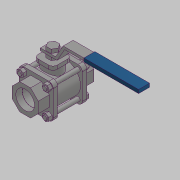
# Autodesk Inventor part: MANUAL THREADED BALL VALVE DN32 S235
Saved by Autodesk Inventor 2017 (Build 210142000, 142)
## iProperties
Created: 2017-11-25
Part Number: MANUAL THREADED BALL VALVE DN32 S235
Material: S235
Document SubType Name: Modeling
Designer: Demarec
Density: 7.85 g/cm^3
Appearance: Plate(1)
Description: BELVEN BV3
Author: Demarec
Autodesk Inventor part; units mm, degrees
ref_plane "YZ Plane" through (0, 0, 0) normal (1, 0, 0) x (0, 1, 0)
ref_plane "XZ Plane" through (0, 0, 0) normal (0, 1, 0) x (-1, 0, 0)
sketch "Sketch3" plane through (0, 0, 0) normal (0, 1, 0) x (-1, 0, 0)
  line L0 (-10.3553, 25) -> (10.3553, 25)
  line L1 (10.3553, 25) -> (25, 10.3553)
  line L2 (25, 10.3553) -> (25, -10.3553)
  line L3 (25, -10.3553) -> (10.3553, -25)
  line L4 (10.3553, -25) -> (-10.3553, -25)
  line L5 (-10.3553, -25) -> (-25, -10.3553)
  line L6 (-25, -10.3553) -> (-25, 10.3553)
  line L7 (-25, 10.3553) -> (-10.3553, 25)
  circle A0 centre (0, 0) radius 27.0598
  line L8 (24.375, -32.5) -> (-24.375, -32.5)
  line L9 (-32.5, -24.375) -> (-32.5, 24.375)
  line L10 (-24.375, 32.5) -> (24.375, 32.5)
  line L11 (32.5, 24.375) -> (32.5, -24.375)
  line L12 (32.5, -32.5) -> (-32.5, 32.5) construction
  line L13 (-32.5, -32.5) -> (32.5, 32.5) construction
  circle A1 centre (0, 0) radius 25
  arc A2 (32.5, 24.375) -> (24.375, 32.5) centre (24.375, 24.375) ccw
  arc A3 (-24.375, 32.5) -> (-32.5, 24.375) centre (-24.375, 24.375) ccw
  arc A4 (-32.5, -24.375) -> (-24.375, -32.5) centre (-24.375, -24.375) ccw
  arc A5 (24.375, -32.5) -> (32.5, -24.375) centre (24.375, -24.375) ccw
  circle A6 centre (0, 0) radius 17.5
  circle A7 centre (24.375, 24.375) radius 4
  circle A8 centre (0, 0) radius 29.0598
  dimension "oSW" = 50
  dimension "oFlangeW" = 65
  dimension "d2" = 8.125
  dimension "oIntDia" = 35
  dimension "oMbolt" = 8
  dimension "d16" = 2
  constraints: 28 end point, 9 tangent, 8 centre point, 8 point on circle, 8 point on line, 5 coincident, 3 equal radius, 2 horizontal, 2 midpoint, 2 parallel, 2 perpendicular, 20 other
  measures "oSW" distance between parallel lines of L6 L2
  measures "oFlangeW" distance of L12.start L13.start
  measures "d2" radius of A2
  measures "oIntDia" diameter of A6
  measures "oMbolt" diameter of A7
extrude "Extrusion1" add sketch "Sketch3" along normal mid plane 106 contours L0 A1 L7 | L0 L1 A1 | A1 | A1 L6 L7 | L1 L2 A1 | A1 L5 L6 | L2 L3 A1 | A1 L4 L5 | L3 L4 A1
extrude "Extrusion2" add sketch "Sketch3" along normal mid plane 64 contours A0 L0 | L7 A0 | A0 L1 | L6 A0 | A0 L2 | L5 A0 | L4 A0 | A0 L3 | L8 A4 L9 A3 L10 A2 L11 A5 | A7 | A8
extrude "Extrusion3" cut sketch "Sketch3" along normal mid plane 47 contours L8 A4 L9 A3 L10 A2 L11 A5 | A7
extrude "Extrusion4" add sketch "Sketch3" along normal mid plane 80 contours A7
sketch "Sketch4" plane through (0, -32, 0) normal (0, -1, 0) x (1, 0, 0)
  circle A0 centre (-24.375, 24.375) radius 4 projected
  line L0 (-20.9109, 18.375) -> (-27.8391, 18.375)
  line L1 (-27.8391, 18.375) -> (-31.3032, 24.375)
  line L2 (-31.3032, 24.375) -> (-27.8391, 30.375)
  line L3 (-27.8391, 30.375) -> (-20.9109, 30.375)
  line L4 (-20.9109, 30.375) -> (-17.4468, 24.375)
  line L5 (-17.4468, 24.375) -> (-20.9109, 18.375)
  point P0 (0, 0)
  dimension "d13" = 12
  constraints: 12 end point, 1 coincident, 1 horizontal, 13 other
  measures "d13" distance between parallel lines of L0 L3
extrude "Extrusion5" add sketch "Sketch4" along normal blind 6.4
sketch "Sketch10" plane through (0, 53, 0) normal (0, 1, 0) x (1, 0, 0)
  circle A0 centre (0, 0) radius 17.5 projected
  circle A1 centre (0, 0) radius 17.75
  dimension "d44" = 0.25
  constraints: 1 centre point
  measures "d44" radial gap between concentric circles of A0 A1
extrude "Extrusion11" cut sketch "Sketch10" against normal blind 12
mirror "Mirror1" about plane through (0, 0, 0) normal (0, 1, 0) of "Extrusion5", "Extrusion11"
pattern_circular "Circular Pattern1" count 4 over 360 about axis through (0, 0, 0) along (0, 1, 0) of "Extrusion5", "Extrusion4", "Mirror1"
ref_plane "Work Plane1" through (0, 0, 45) normal (0, 0, 1) x (1, 0, 0)
sketch "Sketch5" plane through (0, 0, 45) normal (0, 0, 1) x (1, 0, 0)
  line L0 (-9.875, -18) -> (9.875, -18)
  line L1 (18, -9.875) -> (18, 9.875)
  line L2 (9.875, 18) -> (-9.875, 18)
  line L3 (-18, 9.875) -> (-18, -9.875)
  line L4 (-18, -18) -> (18, 18) construction
  line L5 (18, -18) -> (-18, 18) construction
  arc A0 (-18, -9.875) -> (-9.875, -18) centre (-9.875, -9.875) ccw
  arc A1 (9.875, -18) -> (18, -9.875) centre (9.875, -9.875) ccw
  arc A2 (18, 9.875) -> (9.875, 18) centre (9.875, 9.875) ccw
  arc A3 (-9.875, 18) -> (-18, 9.875) centre (-9.875, 9.875) ccw
  point P0 (0, 0)
  dimension "d21" = 36
  dimension "d22" = 8.125
  constraints: 12 end point, 8 point on circle, 8 point on line, 8 tangent, 4 centre point, 3 equal radius, 2 midpoint, 2 parallel, 2 perpendicular, 1 horizontal
  measures "d21" distance of L4.start L5.start
  measures "d22" radius of A0
extrude "Extrusion6" add sketch "Sketch5" against normal blind 7
sketch "Sketch6" plane through (0, 0, 38) normal (0, 0, -1) x (-1, 0, 0)
  circle A0 centre (0, 0) radius 17.5
  dimension "d25" = 35
  constraints: 1 centre point, 1 coincident
  measures "d25" diameter of A0
extrude "Extrusion7" add sketch "Sketch6" along normal up to surface
sketch "Sketch8" plane through (0, 0, 45) normal (0, 0, 1) x (1, 0, 0)
  line L0 (-4.9075, -8.5) -> (-9.815, 0)
  line L1 (-9.815, 0) -> (-4.9075, 8.5)
  line L2 (-4.9075, 8.5) -> (4.9075, 8.5)
  line L3 (4.9075, 8.5) -> (9.815, 0)
  line L4 (9.815, 0) -> (4.9075, -8.5)
  line L5 (4.9075, -8.5) -> (-4.9075, -8.5)
  point P0 (0, 0)
  point P1 (0, 0)
  dimension "oSW2" = 17
  constraints: 12 end point, 1 coincident, 1 horizontal, 13 other
  measures "oSW2" distance between parallel lines of L2 L5
extrude "Extrusion8" add sketch "Sketch8" along normal blind 19
sketch "Sketch9" plane through (0, 0, 0) normal (0, 1, 0) x (-1, 0, 0)
  line L0 (-9.815, 45) -> (-9.815, 64) projected
  line L1 (-14.565, 52.125) -> (17.3074, 52.125)
  line L2 (17.3074, 52.125) -> (31.7411, 77.125)
  line L3 (31.7411, 77.125) -> (69.6, 77.125)
  line L4 (69.6, 77.125) -> (69.6, 81.875)
  line L5 (69.6, 81.875) -> (28.9987, 81.875)
  line L6 (28.9987, 81.875) -> (14.565, 56.875)
  line L7 (14.565, 56.875) -> (-14.565, 56.875)
  line L8 (-14.565, 56.875) -> (-14.565, 52.125)
  line L9 (-9.815, 54.5) -> (-14.565, 54.5) construction
  line L10 (19.8191, 56.4755) -> (15.7055, 58.8505) construction
  line L11 (69.6, 82.875) -> (174, 82.875)
  line L12 (174, 82.875) -> (174, 76.125)
  line L13 (174, 76.125) -> (69.6, 76.125)
  line L14 (69.6, 76.125) -> (69.6, 82.875)
  line L15 (9.815, 45) -> (9.815, 64) projected
  point P0 (0, 0)
  point P1 (69.6, 79.5)
  dimension "d32" = 60
  dimension "d33" = 4.75
  dimension "oHeightHandle" = 25
  dimension "d35" = 1
  dimension "d36" = 4.75
  dimension "d37" = 4.75
  dimension "oLenghtHandle" = 174
  dimension "d39" = 104.4
  constraints: 28 end point, 6 perpendicular, 4 midpoint, 4 parallel, 3 horizontal, 2 equal length, 2 point on line
  measures "d32" angle of L6 L7
  measures "d33" distance of L7.end L1.start
  measures "oHeightHandle" distance between parallel lines of L5 L7
  measures "d35" distance between parallel lines of L11 L5
  measures "d36" distance between parallel lines of L0 L8
  measures "d37" distance from line of L15 L6.end
  measures "oLenghtHandle" distance from line of point (0, 0) L12
  measures "d39" distance of L11.start L11.end
extrude "Extrusion9" add sketch "Sketch9" along normal mid plane 19 contours L1 L8 L7 L0 | L0 L7 L15 L1 | L15 L7 L6 L5 L4 L3 L2 L1
extrude "Extrusion10" add sketch "Sketch9" along normal mid plane 21 contours L4 L14 L11 L12 L13
equation "\"d2\" = 0.125 * oFlangeW"
equation "\"d13\" = 1.5 * oMbolt"
equation "\"d14\" = 0.8 * oMbolt"
equation "\"d22\" = d2"
equation "\"d25\" = oIntDia"
equation "\"d33\" = 0.25 * oHeightTop"
equation "\"d36\" = d33"
equation "\"d37\" = d36"
equation "\"d39\" = 0.6 * oLenghtHandle"
equation "\"oHeightTop\" = 19"
body "Solid1"
